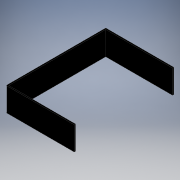
# Autodesk Inventor part: Visor
Saved by Autodesk Inventor 2019 (Build 230136000, 136)
## iProperties
Created: 2020-03-15
Part Number: Visor
Material: Generic
Document SubType Name: Modeling
Designer: james
Density: 1 g/cm^3
Appearance: Default(1)
Author: james
Autodesk Inventor part; units mm, degrees
ref_plane "YZ Plane" through (0, 0, 0) normal (1, 0, 0) x (0, 1, 0)
ref_plane "XZ Plane" through (0, 0, 0) normal (0, 1, 0) x (-1, 0, 0)
ref_plane "XY Plane" through (0, 0, 0) normal (0, 0, 1) x (1, 0, 0)
sketch "Sketch1" plane through (0, 0, 0) normal (0, 1, 0) x (-1, 0, 0)
  line L0 (199.9677, 280.6608) -> (-123.8823, 280.6608)
  line L1 (-123.8823, 280.6608) -> (-123.8823, 287.0108)
  line L2 (-123.8823, 287.0108) -> (206.3177, 287.0108)
  line L3 (206.3177, 287.0108) -> (206.3177, -195.5892)
  line L4 (206.3177, -195.5892) -> (-123.8823, -195.5892)
  line L5 (-123.8823, -195.5892) -> (-123.8823, -189.2392)
  line L6 (-123.8823, -189.2392) -> (199.9677, -189.2392)
  line L7 (199.9677, -189.2392) -> (199.9677, 280.6608)
  point P0 (0, 0)
  dimension "d0" = 482.6
  dimension "d1" = 330.2
  dimension "d2" = 6.35
  dimension "d3" = 6.35
  dimension "d4" = 6.35
  constraints: 16 end point, 6 perpendicular, 2 point on line, 1 horizontal
  measures "d0" distance of L2.end L3.end
  measures "d1" distance of L1.end L2.end
  measures "d2" distance between parallel lines of L7 L3
  measures "d3" distance between parallel lines of L2 L0
  measures "d4" distance between parallel lines of L4 L6
extrude "Extrusion1" add sketch "Sketch1" along normal blind 114.3
fillet "Fillet1" radius 3.175 2 edges at (-206.3177, 57.15, 287.0108) (-206.3177, 57.15, -195.5892)
body "Solid1"
